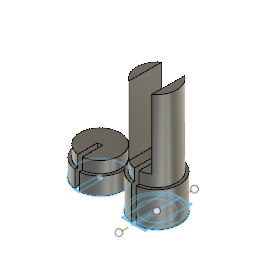
light-jar-frame v3 (Autodesk Fusion 360 design; units mm, degrees)
Autodesk Fusion 360 part; units mm, degrees
sketch "Sketch1" plane through (0, 0, 0) normal (0, 0, 1) x (1, 0, 0)
  circle A0 centre (-54.6636, 37.8571) radius 20
  line L0 (-56.6636, 37.8571) -> (-52.6636, 37.8571)
  line L1 (-52.6636, 37.8571) -> (-52.6636, 17.8571)
  line L2 (-52.6636, 17.8571) -> (-56.6636, 17.8571)
  line L3 (-56.6636, 17.8571) -> (-56.6636, 37.8571)
  line L4 (-6.6636, 37.1429) -> (-2.6636, 37.1429)
  line L5 (-2.6636, 17.1429) -> (-6.6636, 17.1429)
  line L6 (-2.6636, 37.1429) -> (-2.6636, 17.1429)
  line L7 (-6.6636, 17.1429) -> (-6.6636, 37.1429)
  circle A1 centre (-4.6636, 37.1429) radius 20
  circle A2 centre (-4.6636, 37.1429) radius 12.5
  circle A3 centre (-4.6636, 37.1429) radius 17.5
  line L8 (-4.6636, 4.2892) -> (-4.6636, 70) construction
  line L9 (-4.6636, 57.1429) -> (-14.6636, 57.1429)
  line L10 (-14.6636, 57.1429) -> (-14.6636, 17.1429)
  line L11 (-14.6636, 17.1429) -> (-4.6636, 17.1429)
  line L12 (-4.6636, 17.1429) -> (-4.6636, 57.1429)
  line L13 (-4.6636, 57.1429) -> (5.3364, 57.1429)
  line L14 (5.3364, 57.1429) -> (5.3364, 17.1429)
  line L15 (5.3364, 17.1429) -> (-4.6636, 17.1429)
  line L16 (-4.6636, 17.1429) -> (-4.6636, 57.1429)
  dimension "d5" = 40
  dimension "d7" = 4
  dimension "d8" = 20
  dimension "d9" = 2
  dimension "d10" = 40
  dimension "d11" = 4
  dimension "d12" = 20
  dimension "d13" = 2
  dimension "d15" = 25
  dimension "d25" = 35
  dimension "d33" = 10
  dimension "d34" = 40
  dimension "d35" = 10
  dimension "d36" = 40
  constraint horizontal L0
  constraint vertical L1
  constraint horizontal L2
  constraint vertical L3
  constraint horizontal L4
  constraint vertical L6
  constraint horizontal L5
  constraint vertical L7
  constraint concentric A1 A2
  constraint concentric A2 A3
  constraint vertical L8
  constraint horizontal L9
  constraint vertical L10
  constraint horizontal L11
  constraint vertical L12
  constraint coincident A1 L9.start
  constraint coincident L8 L9.start
  constraint horizontal L13
  constraint vertical L14
  constraint horizontal L15
  constraint vertical L16
  measures "d5" diameter of A0
  measures "d7" distance of L0.start L0.end
  measures "d8" distance of L0.start L2.end
  measures "d9" distance of A0.centre L0.end
  measures "d10" diameter of A1
  measures "d11" distance of L4.end L4.start
  measures "d12" distance of L5.end L4.start
  measures "d13" distance of L4.end A1.centre
  measures "d15" diameter of A2
  measures "d25" diameter of A3
  measures "d33" distance of L9.start L9.end
  measures "d34" distance of L9.start L11.end
  measures "d35" distance of L9.start L13.end
  measures "d36" distance of L9.start L11.end
extrude "Extrude2" add sketch "Sketch1" along normal blind 40 contours L4 L7 A2 L10 L12 L16 | L4 L6 A2 L12 L14 L16 | L7 A2 A3 L10 | A2 A3 L12 L14 L16 | A2 A3 L10 L12 L16 | A2 A3 L10 | A2 L10 | L6 A2 A3 L14 | A2 A3 L14 | A2 L14 makes body 1
extrude "Extrude1" add sketch "Sketch1" along normal blind 30 separate body contours L4 L7 A2 L10 L12 L16 | L4 L6 A2 L12 L14 L16 | L7 A2 A3 L10 | A2 A3 L12 L14 L16 | A2 A3 L10 L12 L16 | L7 A1 A3 L10 | A2 A3 L10 | A2 L10 | L6 A2 A3 L14 | A2 A3 L14 | A2 L14 | A1 A3 L12 L14 L16 | A1 A3 L10 L12 L16 | A1 A3 L10 | L6 A1 A3 L14 | A1 A3 L14 makes body 2
extrude "Extrude3" cut sketch "Sketch1" along normal blind 1.2 contours L4 L7 A2 L10 L12 L16 | L4 L6 A2 L12 L14 L16 | A2 L10 | A2 L14 bodies 1 2
extrude "Extrude5" add sketch "Sketch1" along normal blind 15 separate body contours A0 L0 L1 L3 picked at (-55.1019, 44.5094) makes body 3
sketch "Sketch2" plane through (0, 0, 15) normal (0, 0, 1) x (-1, 0, 0)
  arc A0 (52.6636, -17.9574) -> (56.6636, -17.9574) centre (54.6636, -37.8571) ccw
  line L0 (56.6636, -17.9574) -> (56.6636, -37.8571)
  line L1 (56.6636, -37.8571) -> (52.6636, -37.8571)
  line L2 (52.6636, -37.8571) -> (52.6636, -17.9574)
  circle A1 centre (54.6636, -37.8571) radius 17.5
  dimension "d44" = 35
  constraint concentric A0 A1
  measures "d44" diameter of A1
extrude "Extrude6" add sketch "Sketch2" along normal blind 10 contours L0 L1 L2 A1 picked at (54.3097, -43.6797) bodies 3
sketch "Sketch4" plane through (0, 37.8571, 0) normal (0, -1, 0) x (1, 0, 0)
  line L0 (-56.6636, 0) -> (-52.6636, 0)
  line L1 (-52.6636, 0) -> (-52.6636, 25)
  line L2 (-52.6636, 25) -> (-56.6636, 25)
  line L3 (-56.6636, 25) -> (-56.6636, 0)
  line L4 (-54.6636, 0) -> (-54.6636, 6)
  line L5 (-54.6636, 0) -> (-35, 0)
  spline S0 degree 2 poles (-35, 0) (-44.8318, 5.0792) (-54.6636, 6) knots 0 0 0 2.077429 2.077429 2.077429 weights 1 3 1
  dimension "d48" = 6
  constraint midpoint L0 L4.start
  constraint perpendicular L0 L4
  constraint perpendicular L4 L5
  measures "d48" distance of L4.start L4.end
revolve "Revolve1" cut sketch "Sketch4" angle 360 about axis through (-54.6636, 37.8571, 0) along (0, 0, -1) contours L0 L1 L4 L5 S0 | L1 L5 S0 bodies 3
extrude "Extrude7" add sketch "Sketch1" along normal blind 100 contours A2 A3 L10 | A2 L10 | A2 A3 L14 | A2 L14 bodies 1 2
equation "diameter = 40 mm"
equation "topHeight = height - lightSheetHeight - bottomHeight"
equation "bottomHeight = 30 mm"
equation "slotWidth = 4 mm"
equation "d5 = diameter"
equation "d7 = slotWidth"
equation "d8 = diameter / 2"
equation "d9 = slotWidth / 2"
equation "d10 = diameter"
equation "d11 = slotWidth"
equation "d12 = diameter / 2"
equation "d13 = slotWidth / 2"
equation "usbBoardWidth = 25 mm"
equation "d15 = usbBoardWidth"
equation "backSupportWidth = 15 mm"
equation "frontSupportWidth = 5 mm"
equation "lightSheetDiameter = 35 mm"
equation "d25 = lightSheetDiameter"
equation "lightSheetHeight = 80 mm"
equation "height = 125 mm"
equation "lightFormInset = 10 mm"
equation "d29 = bottomHeight"
equation "d31 = bottomHeight + lightFormInset"
equation "d33 = diameter - ( backSupportWidth * 2 )"
equation "d34 = diameter"
equation "d35 = diameter - ( backSupportWidth * 2 )"
equation "d36 = diameter"
equation "supportHeight = height - ( topHeight + bottomHeight + ( lightFormInset * 2 ) )"
equation "d42 = topHeight"
equation "d44 = lightSheetDiameter"
equation "d45 = lightFormInset"
equation "dishDepth = 6 mm"
equation "d48 = dishDepth"
equation "d50 = supportHeight + lightFormInset + bottomHeight"
